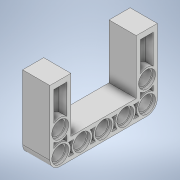
# Autodesk Inventor part: chaimber-adapter
Saved by Autodesk Inventor 2021 (Build 250183000, 183)
## iProperties
Created: 2024-03-14
Part Number: chaimber-adapter
Material: Generic
Document SubType Name: Modeling
Designer: 22hamfri
Density: 1 g/cm^3
Appearance: Default
Author: 22hamfri
Autodesk Inventor part; units mm, degrees
ref_plane "YZ Plane" through (0, 0, 0) normal (1, 0, 0) x (0, 1, 0)
ref_plane "XZ Plane" through (0, 0, 0) normal (0, 1, 0) x (-1, 0, 0)
ref_plane "XY Plane" through (0, 0, 0) normal (0, 0, 1) x (1, 0, 0)
sketch "Sketch1" plane through (0, 0, 0) normal (1, 0, 0) x (0, 1, 0)
  line L0 (0, 0) -> (0, -12)
  line L1 (0, -12) -> (20, -12)
  circle A0 centre (-3.8, 0) radius 3.8
  circle A1 centre (-3.8, 0) radius 3.1
  circle A2 centre (-3.8, 0) radius 2.575
  circle A3 centre (-3.8, -7.97) radius 3.1
  circle A4 centre (-3.8, -7.97) radius 2.575
  circle A5 centre (-3.8, -7.97) radius 3.8
  circle A6 centre (-3.8, -15.94) radius 3.1
  circle A7 centre (-3.8, -15.94) radius 2.575
  circle A8 centre (-3.8, -15.94) radius 3.8
  circle A9 centre (4.17, -15.94) radius 3.8
  circle A10 centre (4.17, -15.94) radius 3.1
  circle A11 centre (4.17, -15.94) radius 2.575
  line L2 (-3.8, -19.74) -> (20, -19.74)
  line L3 (20, -19.74) -> (20, -12)
  line L4 (-7.6, 0) -> (-7.6, -15.94)
  line L5 (-1.225, 0) -> (-6.375, 0)
  line L6 (18, -13.5) -> (18, -18.24)
  line L7 (-0.8869, -13.5) -> (1.2569, -13.5)
  line L8 (7.0831, -13.5) -> (18, -13.5)
  line L9 (-1.5, -3.0249) -> (-1.5, -4.9451)
  line L10 (-1.5, -10.9949) -> (-1.5, -12.9151)
  line L11 (-6.1, -4.9451) -> (-6.1, -3.0249)
  line L12 (-6.1, -12.9151) -> (-6.1, -10.9949)
  line L13 (18, -18.24) -> (7.1949, -18.24)
  line L14 (1.1451, -18.24) -> (-0.7751, -18.24)
  line L15 (0, 0) -> (0, 12)
  line L16 (0, 12) -> (20, 12)
  circle A12 centre (-3.8, 0) radius 3.8
  circle A13 centre (-3.8, 0) radius 3.1
  circle A14 centre (-3.8, 0) radius 2.575
  circle A15 centre (-3.8, 7.97) radius 3.1
  circle A16 centre (-3.8, 7.97) radius 2.575
  circle A17 centre (-3.8, 7.97) radius 3.8
  circle A18 centre (-3.8, 15.94) radius 3.1
  circle A19 centre (-3.8, 15.94) radius 2.575
  circle A20 centre (-3.8, 15.94) radius 3.8
  circle A21 centre (4.17, 15.94) radius 3.8
  circle A22 centre (4.17, 15.94) radius 3.1
  circle A23 centre (4.17, 15.94) radius 2.575
  line L17 (-3.8, 19.74) -> (20, 19.74)
  line L18 (20, 19.74) -> (20, 12)
  line L19 (-7.6, 0) -> (-7.6, 15.94)
  line L20 (18, 13.5) -> (18, 18.24)
  line L21 (-0.8869, 13.5) -> (1.2569, 13.5)
  line L22 (7.0831, 13.5) -> (18, 13.5)
  line L23 (-1.5, 3.0249) -> (-1.5, 4.9451)
  line L24 (-1.5, 10.9949) -> (-1.5, 12.9151)
  line L25 (-6.1, 4.9451) -> (-6.1, 3.0249)
  line L26 (-6.1, 12.9151) -> (-6.1, 10.9949)
  line L27 (18, 18.24) -> (7.1949, 18.24)
  line L28 (1.1451, 18.24) -> (-0.7751, 18.24)
  dimension "d0" = 5.15
  dimension "d1" = 6.2
  dimension "d2" = 0.7
  dimension "d5" = 7.97
  dimension "d12" = 7.97
  dimension "d17" = 20
  dimension "d18" = 2
  dimension "d23" = 1.5
  dimension "d24" = 1.5
  dimension "d25" = 1.5
  dimension "d26" = 1.5
  dimension "d27" = 24
  constraints: 58 end point, 36 point on circle, 24 centre point, 24 symmetric about line, 10 perpendicular, 4 collinear, 4 tangent, 4 vertical, 3 parallel, 2 horizontal, 1 horizontal alignment, 24 other
  measures "d0" diameter of A2
  measures "d1" diameter of A1
  measures "d2" radial gap between concentric circles of A1 A0
  measures "d5" distance of A1.centre A3.centre
  measures "d12" distance of A6.centre A10.centre
  measures "d17" distance between parallel lines of L0 L3
  measures "d18" distance between parallel lines of L3 L6
  measures "d23" distance between parallel lines of L2 L13
  measures "d24" distance between parallel lines of L8 L1
  measures "d25" distance between parallel lines of L0 L10
  measures "d26" distance between parallel lines of L4 L12
  measures "d27" distance between parallel lines of L1 L16
extrude "Extrusion1" add sketch "Sketch1" along normal mid plane 10 contours A0 | L0 A5 L9 A0 | A0 L23 A17 L15 | A5 | L0 L1 L3 L2 A9 L13 L6 L8 L7 A8 L10 A5 | A17 L24 A20 L21 A21 L22 L20 L27 L17 L18 L16 L15 | A17 | A0 L19 A17 L25 | L11 A5 L4 A0 | L12 A8 L4 A5 | A8 | A17 L19 A20 L26 | A20 | L2 A8 L14 A9 | A9 | A21 | A21 L28 A20 L17
extrude "Extrusion2" add sketch "Sketch1" along normal mid plane 8 contours A1 | A3 | A6 | A10 | A15 | A18 | A22
extrude "Extrusion3" add sketch "Sketch1" along normal mid plane 4 contours A0 L25 A17 L23 | L9 A5 L11 A0 | L10 A8 L12 A5 | A17 L26 A20 L24 | L7 A9 L14 A8 | A20 L28 A21 L21 | A9 L8 L6 L13 | L27 L20 L22 A21
equation "\"d24\" = d23"
equation "\"d25\" = d23"
equation "\"d26\" = d23"
equation "\"d20\" = d19"
equation "\"d21\" = d19"
equation "\"d22\" = d19"
equation "\"d19\" = 1.5"
body "Solid1"
